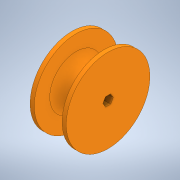
# Autodesk Inventor part: WheelForHangingAndMoving
Saved by Autodesk Inventor 2020.2 (Build 242310000, 310)
## iProperties
Created: 2020-01-06
Part Number: WheelForHangingAndMoving
Material: PBT Plastic
Document SubType Name: Modeling
Designer: steele
Density: 1.31 g/cm^3
Appearance: Orange
Author: steele
Autodesk Inventor part; units mm, degrees
ref_plane "YZ Plane" through (0, 0, 0) normal (1, 0, 0) x (0, 1, 0)
ref_plane "XZ Plane" through (0, 0, 0) normal (0, 1, 0) x (-1, 0, 0)
ref_plane "XY Plane" through (0, 0, 0) normal (0, 0, 1) x (1, 0, 0)
sketch "Sketch1" plane through (0, 0, 0) normal (0, 0, 1) x (1, 0, 0)
  arc A0 (-21.082, 40.132) -> (21.082, 40.132) centre (0, 40.132) ccw
  line L0 (-21.082, 40.132) -> (-21.082, 0)
  line L1 (21.082, 40.132) -> (21.082, 0)
  line L2 (-21.082, 0) -> (21.082, 0)
  line L3 (-21.082, 0) -> (-27.432, 0)
  line L4 (-27.432, 0) -> (-27.432, 63.5)
  line L5 (-27.432, 63.5) -> (-21.082, 63.5)
  line L6 (-21.082, 63.5) -> (-21.082, 0)
  line L7 (21.082, 0) -> (27.432, 0)
  line L8 (27.432, 0) -> (27.432, 63.5)
  line L9 (27.432, 63.5) -> (21.082, 63.5)
  line L10 (21.082, 63.5) -> (21.082, 0)
  point P0 (0, 0)
  dimension "diameterOfPipe" = 42.164
  dimension "d6" = 6.35
  dimension "d7" = 63.5
  dimension "d8" = 6.35
  dimension "d9" = 63.5
  dimension "d13" = 19.05
  constraints: 22 end point, 4 parallel, 3 horizontal, 2 perpendicular, 2 point on circle, 2 vertical, 1 centre point, 1 tangent
  measures "diameterOfPipe" diameter of A0
  measures "d6" distance of L4.end L5.end
  measures "d7" distance of L3.end L4.end
  measures "d8" distance of L9.end L8.end
  measures "d9" distance of L8.end L7.end
  measures "d13" distance edge to line of A0 L2
revolve "Revolution1" add sketch "Sketch1" angle 360 about axis through (-21.082, 0, 0) along (1, 0, 0)
sketch "Sketch3" plane through (27.432, 0, 0) normal (1, 0, 0) x (0, 0, -1)
  line L0 (7.9189, 0) -> (3.9595, -6.858)
  line L1 (3.9595, -6.858) -> (-3.9595, -6.858)
  line L2 (-3.9595, -6.858) -> (-7.9189, 0)
  line L3 (-7.9189, 0) -> (-3.9595, 6.858)
  line L4 (-3.9595, 6.858) -> (3.9595, 6.858)
  line L5 (3.9595, 6.858) -> (7.9189, 0)
  point P0 (0, 0)
  point P1 (0, 0)
  dimension "hexWidth" = 13.716
  constraints: 12 end point, 1 coincident, 1 horizontal, 13 other
  measures "hexWidth" distance between parallel lines of L1 L4
extrude "Extrusion2" cut sketch "Sketch3" against normal through all
equation "\"d6\" = widthOfOutside"
equation "\"d8\" = widthOfOutside"
equation "\"widthOfOutside\" = 6.35"
body "Solid1"
